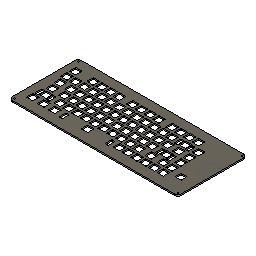
middle (Autodesk Fusion 360 design; units mm, degrees)
part number: 2026-03-14-23-22-41-149
Autodesk Fusion 360 part; units mm, degrees
(part 1 of 2)
sketch "Sketch1" plane through (0, 0, 0) normal (0, 0, 1) x (1, 0, 0)
  line L0 (-139.2143, 66.4682) -> (-126.2143, 66.4682)
  line L1 (-139.2143, 52.4682) -> (-126.2143, 52.4682)
  line L2 (-139.7143, 65.9682) -> (-139.7143, 52.9682)
  line L3 (-125.7143, 65.9682) -> (-125.7143, 52.9682)
  arc A0 (-139.2143, 66.4682) -> (-139.7143, 65.9682) centre (-139.2143, 65.9682) ccw
  arc A1 (-125.7143, 65.9682) -> (-126.2143, 66.4682) centre (-126.2143, 65.9682) ccw
  arc A2 (-139.7143, 52.9682) -> (-139.2143, 52.4682) centre (-139.2143, 52.9682) ccw
  arc A3 (-126.2143, 52.4682) -> (-125.7143, 52.9682) centre (-126.2143, 52.9682) ccw
  line L4 (-101.1143, 66.4682) -> (-88.1143, 66.4682)
  line L5 (-101.1143, 52.4682) -> (-88.1143, 52.4682)
  line L6 (-101.6143, 65.9682) -> (-101.6143, 52.9682)
  line L7 (-87.6143, 65.9682) -> (-87.6143, 52.9682)
  arc A4 (-101.1143, 66.4682) -> (-101.6143, 65.9682) centre (-101.1143, 65.9682) ccw
  arc A5 (-87.6143, 65.9682) -> (-88.1143, 66.4682) centre (-88.1143, 65.9682) ccw
  arc A6 (-101.6143, 52.9682) -> (-101.1143, 52.4682) centre (-101.1143, 52.9682) ccw
  arc A7 (-88.1143, 52.4682) -> (-87.6143, 52.9682) centre (-88.1143, 52.9682) ccw
  line L8 (-82.0643, 66.4682) -> (-69.0643, 66.4682)
  line L9 (-82.0643, 52.4682) -> (-69.0643, 52.4682)
  line L10 (-82.5643, 65.9682) -> (-82.5643, 52.9682)
  line L11 (-68.5643, 65.9682) -> (-68.5643, 52.9682)
  arc A8 (-82.0643, 66.4682) -> (-82.5643, 65.9682) centre (-82.0643, 65.9682) ccw
  arc A9 (-68.5643, 65.9682) -> (-69.0643, 66.4682) centre (-69.0643, 65.9682) ccw
  arc A10 (-82.5643, 52.9682) -> (-82.0643, 52.4682) centre (-82.0643, 52.9682) ccw
  arc A11 (-69.0643, 52.4682) -> (-68.5643, 52.9682) centre (-69.0643, 52.9682) ccw
  line L12 (-63.0143, 66.4682) -> (-50.0143, 66.4682)
  line L13 (-63.0143, 52.4682) -> (-50.0143, 52.4682)
  line L14 (-63.5143, 65.9682) -> (-63.5143, 52.9682)
  line L15 (-49.5143, 65.9682) -> (-49.5143, 52.9682)
  arc A12 (-63.0143, 66.4682) -> (-63.5143, 65.9682) centre (-63.0143, 65.9682) ccw
  arc A13 (-49.5143, 65.9682) -> (-50.0143, 66.4682) centre (-50.0143, 65.9682) ccw
  arc A14 (-63.5143, 52.9682) -> (-63.0143, 52.4682) centre (-63.0143, 52.9682) ccw
  arc A15 (-50.0143, 52.4682) -> (-49.5143, 52.9682) centre (-50.0143, 52.9682) ccw
  line L16 (-43.9643, 66.4682) -> (-30.9643, 66.4682)
  line L17 (-43.9643, 52.4682) -> (-30.9643, 52.4682)
  line L18 (-44.4643, 65.9682) -> (-44.4643, 52.9682)
  line L19 (-30.4643, 65.9682) -> (-30.4643, 52.9682)
  arc A16 (-43.9643, 66.4682) -> (-44.4643, 65.9682) centre (-43.9643, 65.9682) ccw
  arc A17 (-30.4643, 65.9682) -> (-30.9643, 66.4682) centre (-30.9643, 65.9682) ccw
  arc A18 (-44.4643, 52.9682) -> (-43.9643, 52.4682) centre (-43.9643, 52.9682) ccw
  arc A19 (-30.9643, 52.4682) -> (-30.4643, 52.9682) centre (-30.9643, 52.9682) ccw
  line L20 (-15.3893, 66.4682) -> (-2.3893, 66.4682)
  line L21 (-15.3893, 52.4682) -> (-2.3893, 52.4682)
  line L22 (-15.8893, 65.9682) -> (-15.8893, 52.9682)
  line L23 (-1.8893, 65.9682) -> (-1.8893, 52.9682)
  arc A20 (-15.3893, 66.4682) -> (-15.8893, 65.9682) centre (-15.3893, 65.9682) ccw
  arc A21 (-1.8893, 65.9682) -> (-2.3893, 66.4682) centre (-2.3893, 65.9682) ccw
  arc A22 (-15.8893, 52.9682) -> (-15.3893, 52.4682) centre (-15.3893, 52.9682) ccw
  arc A23 (-2.3893, 52.4682) -> (-1.8893, 52.9682) centre (-2.3893, 52.9682) ccw
  line L24 (3.6607, 66.4682) -> (16.6607, 66.4682)
  line L25 (3.6607, 52.4682) -> (16.6607, 52.4682)
  line L26 (3.1607, 65.9682) -> (3.1607, 52.9682)
  line L27 (17.1607, 65.9682) -> (17.1607, 52.9682)
  arc A24 (3.6607, 66.4682) -> (3.1607, 65.9682) centre (3.6607, 65.9682) ccw
  arc A25 (17.1607, 65.9682) -> (16.6607, 66.4682) centre (16.6607, 65.9682) ccw
  arc A26 (3.1607, 52.9682) -> (3.6607, 52.4682) centre (3.6607, 52.9682) ccw
  arc A27 (16.6607, 52.4682) -> (17.1607, 52.9682) centre (16.6607, 52.9682) ccw
  line L28 (22.7107, 66.4682) -> (35.7107, 66.4682)
  line L29 (22.7107, 52.4682) -> (35.7107, 52.4682)
  line L30 (22.2107, 65.9682) -> (22.2107, 52.9682)
  line L31 (36.2107, 65.9682) -> (36.2107, 52.9682)
  arc A28 (22.7107, 66.4682) -> (22.2107, 65.9682) centre (22.7107, 65.9682) ccw
  arc A29 (36.2107, 65.9682) -> (35.7107, 66.4682) centre (35.7107, 65.9682) ccw
  arc A30 (22.2107, 52.9682) -> (22.7107, 52.4682) centre (22.7107, 52.9682) ccw
  arc A31 (35.7107, 52.4682) -> (36.2107, 52.9682) centre (35.7107, 52.9682) ccw
  line L32 (41.7607, 66.4682) -> (54.7607, 66.4682)
  line L33 (41.7607, 52.4682) -> (54.7607, 52.4682)
  line L34 (41.2607, 65.9682) -> (41.2607, 52.9682)
  line L35 (55.2607, 65.9682) -> (55.2607, 52.9682)
  arc A32 (41.7607, 66.4682) -> (41.2607, 65.9682) centre (41.7607, 65.9682) ccw
  arc A33 (55.2607, 65.9682) -> (54.7607, 66.4682) centre (54.7607, 65.9682) ccw
  arc A34 (41.2607, 52.9682) -> (41.7607, 52.4682) centre (41.7607, 52.9682) ccw
  arc A35 (54.7607, 52.4682) -> (55.2607, 52.9682) centre (54.7607, 52.9682) ccw
  line L36 (70.3357, 66.4682) -> (83.3357, 66.4682)
  line L37 (70.3357, 52.4682) -> (83.3357, 52.4682)
  line L38 (69.8357, 65.9682) -> (69.8357, 52.9682)
  line L39 (83.8357, 65.9682) -> (83.8357, 52.9682)
  arc A36 (70.3357, 66.4682) -> (69.8357, 65.9682) centre (70.3357, 65.9682) ccw
  arc A37 (83.8357, 65.9682) -> (83.3357, 66.4682) centre (83.3357, 65.9682) ccw
  arc A38 (69.8357, 52.9682) -> (70.3357, 52.4682) centre (70.3357, 52.9682) ccw
  arc A39 (83.3357, 52.4682) -> (83.8357, 52.9682) centre (83.3357, 52.9682) ccw
  line L40 (89.3857, 66.4682) -> (102.3857, 66.4682)
  line L41 (89.3857, 52.4682) -> (102.3857, 52.4682)
  line L42 (88.8857, 65.9682) -> (88.8857, 52.9682)
  line L43 (102.8857, 65.9682) -> (102.8857, 52.9682)
  arc A40 (89.3857, 66.4682) -> (88.8857, 65.9682) centre (89.3857, 65.9682) ccw
  arc A41 (102.8857, 65.9682) -> (102.3857, 66.4682) centre (102.3857, 65.9682) ccw
  arc A42 (88.8857, 52.9682) -> (89.3857, 52.4682) centre (89.3857, 52.9682) ccw
  arc A43 (102.3857, 52.4682) -> (102.8857, 52.9682) centre (102.3857, 52.9682) ccw
  line L44 (108.4357, 66.4682) -> (121.4357, 66.4682)
  line L45 (108.4357, 52.4682) -> (121.4357, 52.4682)
  line L46 (107.9357, 65.9682) -> (107.9357, 52.9682)
  line L47 (121.9357, 65.9682) -> (121.9357, 52.9682)
  arc A44 (108.4357, 66.4682) -> (107.9357, 65.9682) centre (108.4357, 65.9682) ccw
  arc A45 (121.9357, 65.9682) -> (121.4357, 66.4682) centre (121.4357, 65.9682) ccw
  arc A46 (107.9357, 52.9682) -> (108.4357, 52.4682) centre (108.4357, 52.9682) ccw
  arc A47 (121.4357, 52.4682) -> (121.9357, 52.9682) centre (121.4357, 52.9682) ccw
  line L48 (127.4857, 66.4682) -> (140.4857, 66.4682)
  line L49 (127.4857, 52.4682) -> (140.4857, 52.4682)
  line L50 (126.9857, 65.9682) -> (126.9857, 52.9682)
  line L51 (140.9857, 65.9682) -> (140.9857, 52.9682)
  arc A48 (127.4857, 66.4682) -> (126.9857, 65.9682) centre (127.4857, 65.9682) ccw
  arc A49 (140.9857, 65.9682) -> (140.4857, 66.4682) centre (140.4857, 65.9682) ccw
  arc A50 (126.9857, 52.9682) -> (127.4857, 52.4682) centre (127.4857, 52.9682) ccw
  arc A51 (140.4857, 52.4682) -> (140.9857, 52.9682) centre (140.4857, 52.9682) ccw
  line L52 (-139.2143, 47.4182) -> (-126.2143, 47.4182)
  line L53 (-139.2143, 33.4182) -> (-126.2143, 33.4182)
  line L54 (-139.7143, 46.9182) -> (-139.7143, 33.9182)
  line L55 (-125.7143, 46.9182) -> (-125.7143, 33.9182)
  arc A52 (-139.2143, 47.4182) -> (-139.7143, 46.9182) centre (-139.2143, 46.9182) ccw
  arc A53 (-125.7143, 46.9182) -> (-126.2143, 47.4182) centre (-126.2143, 46.9182) ccw
  arc A54 (-139.7143, 33.9182) -> (-139.2143, 33.4182) centre (-139.2143, 33.9182) ccw
  arc A55 (-126.2143, 33.4182) -> (-125.7143, 33.9182) centre (-126.2143, 33.9182) ccw
  line L56 (-120.1643, 47.4182) -> (-107.1643, 47.4182)
  line L57 (-120.1643, 33.4182) -> (-107.1643, 33.4182)
  line L58 (-120.6643, 46.9182) -> (-120.6643, 33.9182)
  line L59 (-106.6643, 46.9182) -> (-106.6643, 33.9182)
  arc A56 (-120.1643, 47.4182) -> (-120.6643, 46.9182) centre (-120.1643, 46.9182) ccw
  arc A57 (-106.6643, 46.9182) -> (-107.1643, 47.4182) centre (-107.1643, 46.9182) ccw
  arc A58 (-120.6643, 33.9182) -> (-120.1643, 33.4182) centre (-120.1643, 33.9182) ccw
  arc A59 (-107.1643, 33.4182) -> (-106.6643, 33.9182) centre (-107.1643, 33.9182) ccw
  line L60 (-101.1143, 47.4182) -> (-88.1143, 47.4182)
  line L61 (-101.1143, 33.4182) -> (-88.1143, 33.4182)
  line L62 (-101.6143, 46.9182) -> (-101.6143, 33.9182)
  line L63 (-87.6143, 46.9182) -> (-87.6143, 33.9182)
  arc A60 (-101.1143, 47.4182) -> (-101.6143, 46.9182) centre (-101.1143, 46.9182) ccw
  arc A61 (-87.6143, 46.9182) -> (-88.1143, 47.4182) centre (-88.1143, 46.9182) ccw
  arc A62 (-101.6143, 33.9182) -> (-101.1143, 33.4182) centre (-101.1143, 33.9182) ccw
  arc A63 (-88.1143, 33.4182) -> (-87.6143, 33.9182) centre (-88.1143, 33.9182) ccw
  line L64 (-82.0643, 47.4182) -> (-69.0643, 47.4182)
  line L65 (-82.0643, 33.4182) -> (-69.0643, 33.4182)
  line L66 (-82.5643, 46.9182) -> (-82.5643, 33.9182)
  line L67 (-68.5643, 46.9182) -> (-68.5643, 33.9182)
  arc A64 (-82.0643, 47.4182) -> (-82.5643, 46.9182) centre (-82.0643, 46.9182) ccw
  arc A65 (-68.5643, 46.9182) -> (-69.0643, 47.4182) centre (-69.0643, 46.9182) ccw
  arc A66 (-82.5643, 33.9182) -> (-82.0643, 33.4182) centre (-82.0643, 33.9182) ccw
  arc A67 (-69.0643, 33.4182) -> (-68.5643, 33.9182) centre (-69.0643, 33.9182) ccw
  line L68 (-63.0143, 47.4182) -> (-50.0143, 47.4182)
  line L69 (-63.0143, 33.4182) -> (-50.0143, 33.4182)
  line L70 (-63.5143, 46.9182) -> (-63.5143, 33.9182)
  line L71 (-49.5143, 46.9182) -> (-49.5143, 33.9182)
  arc A68 (-63.0143, 47.4182) -> (-63.5143, 46.9182) centre (-63.0143, 46.9182) ccw
  arc A69 (-49.5143, 46.9182) -> (-50.0143, 47.4182) centre (-50.0143, 46.9182) ccw
  arc A70 (-63.5143, 33.9182) -> (-63.0143, 33.4182) centre (-63.0143, 33.9182) ccw
  arc A71 (-50.0143, 33.4182) -> (-49.5143, 33.9182) centre (-50.0143, 33.9182) ccw
  line L72 (-43.9643, 47.4182) -> (-30.9643, 47.4182)
  line L73 (-43.9643, 33.4182) -> (-30.9643, 33.4182)
  line L74 (-44.4643, 46.9182) -> (-44.4643, 33.9182)
  line L75 (-30.4643, 46.9182) -> (-30.4643, 33.9182)
  arc A72 (-43.9643, 47.4182) -> (-44.4643, 46.9182) centre (-43.9643, 46.9182) ccw
  arc A73 (-30.4643, 46.9182) -> (-30.9643, 47.4182) centre (-30.9643, 46.9182) ccw
  arc A74 (-44.4643, 33.9182) -> (-43.9643, 33.4182) centre (-43.9643, 33.9182) ccw
  arc A75 (-30.9643, 33.4182) -> (-30.4643, 33.9182) centre (-30.9643, 33.9182) ccw
  line L76 (-24.9143, 47.4182) -> (-11.9143, 47.4182)
  line L77 (-24.9143, 33.4182) -> (-11.9143, 33.4182)
  line L78 (-25.4143, 46.9182) -> (-25.4143, 33.9182)
  line L79 (-11.4143, 46.9182) -> (-11.4143, 33.9182)
  arc A76 (-24.9143, 47.4182) -> (-25.4143, 46.9182) centre (-24.9143, 46.9182) ccw
  arc A77 (-11.4143, 46.9182) -> (-11.9143, 47.4182) centre (-11.9143, 46.9182) ccw
  arc A78 (-25.4143, 33.9182) -> (-24.9143, 33.4182) centre (-24.9143, 33.9182) ccw
  arc A79 (-11.9143, 33.4182) -> (-11.4143, 33.9182) centre (-11.9143, 33.9182) ccw
  line L80 (-5.8643, 47.4182) -> (7.1357, 47.4182)
  line L81 (-5.8643, 33.4182) -> (7.1357, 33.4182)
  line L82 (-6.3643, 46.9182) -> (-6.3643, 33.9182)
  line L83 (7.6357, 46.9182) -> (7.6357, 33.9182)
  arc A80 (-5.8643, 47.4182) -> (-6.3643, 46.9182) centre (-5.8643, 46.9182) ccw
  arc A81 (7.6357, 46.9182) -> (7.1357, 47.4182) centre (7.1357, 46.9182) ccw
  arc A82 (-6.3643, 33.9182) -> (-5.8643, 33.4182) centre (-5.8643, 33.9182) ccw
  arc A83 (7.1357, 33.4182) -> (7.6357, 33.9182) centre (7.1357, 33.9182) ccw
  line L84 (13.1857, 47.4182) -> (26.1857, 47.4182)
  line L85 (13.1857, 33.4182) -> (26.1857, 33.4182)
  line L86 (12.6857, 46.9182) -> (12.6857, 33.9182)
  line L87 (26.6857, 46.9182) -> (26.6857, 33.9182)
  arc A84 (13.1857, 47.4182) -> (12.6857, 46.9182) centre (13.1857, 46.9182) ccw
  arc A85 (26.6857, 46.9182) -> (26.1857, 47.4182) centre (26.1857, 46.9182) ccw
  arc A86 (12.6857, 33.9182) -> (13.1857, 33.4182) centre (13.1857, 33.9182) ccw
  arc A87 (26.1857, 33.4182) -> (26.6857, 33.9182) centre (26.1857, 33.9182) ccw
  line L88 (32.2357, 47.4182) -> (45.2357, 47.4182)
  line L89 (32.2357, 33.4182) -> (45.2357, 33.4182)
  line L90 (31.7357, 46.9182) -> (31.7357, 33.9182)
  line L91 (45.7357, 46.9182) -> (45.7357, 33.9182)
  arc A88 (32.2357, 47.4182) -> (31.7357, 46.9182) centre (32.2357, 46.9182) ccw
  arc A89 (45.7357, 46.9182) -> (45.2357, 47.4182) centre (45.2357, 46.9182) ccw
  arc A90 (31.7357, 33.9182) -> (32.2357, 33.4182) centre (32.2357, 33.9182) ccw
  arc A91 (45.2357, 33.4182) -> (45.7357, 33.9182) centre (45.2357, 33.9182) ccw
  line L92 (51.2857, 47.4182) -> (64.2857, 47.4182)
  line L93 (51.2857, 33.4182) -> (64.2857, 33.4182)
  line L94 (50.7857, 46.9182) -> (50.7857, 33.9182)
  line L95 (64.7857, 46.9182) -> (64.7857, 33.9182)
  arc A92 (51.2857, 47.4182) -> (50.7857, 46.9182) centre (51.2857, 46.9182) ccw
  arc A93 (64.7857, 46.9182) -> (64.2857, 47.4182) centre (64.2857, 46.9182) ccw
  arc A94 (50.7857, 33.9182) -> (51.2857, 33.4182) centre (51.2857, 33.9182) ccw
  arc A95 (64.2857, 33.4182) -> (64.7857, 33.9182) centre (64.2857, 33.9182) ccw
  line L96 (70.3357, 47.4182) -> (83.3357, 47.4182)
  line L97 (70.3357, 33.4182) -> (83.3357, 33.4182)
  line L98 (69.8357, 46.9182) -> (69.8357, 33.9182)
  line L99 (83.8357, 46.9182) -> (83.8357, 33.9182)
  arc A96 (70.3357, 47.4182) -> (69.8357, 46.9182) centre (70.3357, 46.9182) ccw
  arc A97 (83.8357, 46.9182) -> (83.3357, 47.4182) centre (83.3357, 46.9182) ccw
  arc A98 (69.8357, 33.9182) -> (70.3357, 33.4182) centre (70.3357, 33.9182) ccw
  arc A99 (83.3357, 33.4182) -> (83.8357, 33.9182) centre (83.3357, 33.9182) ccw
  line L100 (89.3857, 47.4182) -> (102.3857, 47.4182)
  line L101 (89.3857, 33.4182) -> (102.3857, 33.4182)
  line L102 (88.8857, 46.9182) -> (88.8857, 33.9182)
  line L103 (102.8857, 46.9182) -> (102.8857, 33.9182)
  arc A100 (89.3857, 47.4182) -> (88.8857, 46.9182) centre (89.3857, 46.9182) ccw
  arc A101 (102.8857, 46.9182) -> (102.3857, 47.4182) centre (102.3857, 46.9182) ccw
  arc A102 (88.8857, 33.9182) -> (89.3857, 33.4182) centre (89.3857, 33.9182) ccw
  arc A103 (102.3857, 33.4182) -> (102.8857, 33.9182) centre (102.3857, 33.9182) ccw
  line L104 (117.9607, 47.4182) -> (130.9607, 47.4182)
  line L105 (117.9607, 33.4182) -> (130.9607, 33.4182)
  line L106 (117.4607, 46.9182) -> (117.4607, 33.9182)
  line L107 (131.4607, 46.9182) -> (131.4607, 33.9182)
  arc A104 (117.9607, 47.4182) -> (117.4607, 46.9182) centre (117.9607, 46.9182) ccw
  arc A105 (131.4607, 46.9182) -> (130.9607, 47.4182) centre (130.9607, 46.9182) ccw
  arc A106 (117.4607, 33.9182) -> (117.9607, 33.4182) centre (117.9607, 33.9182) ccw
  arc A107 (130.9607, 33.4182) -> (131.4607, 33.9182) centre (130.9607, 33.9182) ccw
  line L108 (109.5227, 46.4182) -> (115.5227, 46.4182)
  line L109 (109.5227, 31.4182) -> (115.5227, 31.4182)
  line L110 (109.0227, 45.9182) -> (109.0227, 31.9182)
  line L111 (116.0227, 45.9182) -> (116.0227, 31.9182)
  arc A108 (109.5227, 46.4182) -> (109.0227, 45.9182) centre (109.5227, 45.9182) ccw
  arc A109 (116.0227, 45.9182) -> (115.5227, 46.4182) centre (115.5227, 45.9182) ccw
  arc A110 (109.0227, 31.9182) -> (109.5227, 31.4182) centre (109.5227, 31.9182) ccw
  arc A111 (115.5227, 31.4182) -> (116.0227, 31.9182) centre (115.5227, 31.9182) ccw
  line L112 (133.3987, 46.4182) -> (139.3987, 46.4182)
  line L113 (133.3987, 31.4182) -> (139.3987, 31.4182)
  line L114 (132.8987, 45.9182) -> (132.8987, 31.9182)
  line L115 (139.8987, 45.9182) -> (139.8987, 31.9182)
  arc A112 (133.3987, 46.4182) -> (132.8987, 45.9182) centre (133.3987, 45.9182) ccw
  arc A113 (139.8987, 45.9182) -> (139.3987, 46.4182) centre (139.3987, 45.9182) ccw
  arc A114 (132.8987, 31.9182) -> (133.3987, 31.4182) centre (133.3987, 31.9182) ccw
  arc A115 (139.3987, 31.4182) -> (139.8987, 31.9182) centre (139.3987, 31.9182) ccw
  line L116 (146.5357, 47.4182) -> (159.5357, 47.4182)
  line L117 (146.5357, 33.4182) -> (159.5357, 33.4182)
  line L118 (146.0357, 46.9182) -> (146.0357, 33.9182)
  line L119 (160.0357, 46.9182) -> (160.0357, 33.9182)
  arc A116 (146.5357, 47.4182) -> (146.0357, 46.9182) centre (146.5357, 46.9182) ccw
  arc A117 (160.0357, 46.9182) -> (159.5357, 47.4182) centre (159.5357, 46.9182) ccw
  arc A118 (146.0357, 33.9182) -> (146.5357, 33.4182) centre (146.5357, 33.9182) ccw
  arc A119 (159.5357, 33.4182) -> (160.0357, 33.9182) centre (159.5357, 33.9182) ccw
  line L120 (-134.4518, 28.3682) -> (-121.4518, 28.3682)
  line L121 (-134.4518, 14.3682) -> (-121.4518, 14.3682)
  line L122 (-134.9518, 27.8682) -> (-134.9518, 14.8682)
  line L123 (-120.9518, 27.8682) -> (-120.9518, 14.8682)
  arc A120 (-134.4518, 28.3682) -> (-134.9518, 27.8682) centre (-134.4518, 27.8682) ccw
  arc A121 (-120.9518, 27.8682) -> (-121.4518, 28.3682) centre (-121.4518, 27.8682) ccw
  arc A122 (-134.9518, 14.8682) -> (-134.4518, 14.3682) centre (-134.4518, 14.8682) ccw
  arc A123 (-121.4518, 14.3682) -> (-120.9518, 14.8682) centre (-121.4518, 14.8682) ccw
  line L124 (-110.6393, 28.3682) -> (-97.6393, 28.3682)
  line L125 (-110.6393, 14.3682) -> (-97.6393, 14.3682)
  line L126 (-111.1393, 27.8682) -> (-111.1393, 14.8682)
  line L127 (-97.1393, 27.8682) -> (-97.1393, 14.8682)
  arc A124 (-110.6393, 28.3682) -> (-111.1393, 27.8682) centre (-110.6393, 27.8682) ccw
  arc A125 (-97.1393, 27.8682) -> (-97.6393, 28.3682) centre (-97.6393, 27.8682) ccw
  arc A126 (-111.1393, 14.8682) -> (-110.6393, 14.3682) centre (-110.6393, 14.8682) ccw
  arc A127 (-97.6393, 14.3682) -> (-97.1393, 14.8682) centre (-97.6393, 14.8682) ccw
  line L128 (-91.5893, 28.3682) -> (-78.5893, 28.3682)
  line L129 (-91.5893, 14.3682) -> (-78.5893, 14.3682)
  line L130 (-92.0893, 27.8682) -> (-92.0893, 14.8682)
  line L131 (-78.0893, 27.8682) -> (-78.0893, 14.8682)
  arc A128 (-91.5893, 28.3682) -> (-92.0893, 27.8682) centre (-91.5893, 27.8682) ccw
  arc A129 (-78.0893, 27.8682) -> (-78.5893, 28.3682) centre (-78.5893, 27.8682) ccw
  arc A130 (-92.0893, 14.8682) -> (-91.5893, 14.3682) centre (-91.5893, 14.8682) ccw
  arc A131 (-78.5893, 14.3682) -> (-78.0893, 14.8682) centre (-78.5893, 14.8682) ccw
  line L132 (-72.5393, 28.3682) -> (-59.5393, 28.3682)
  line L133 (-72.5393, 14.3682) -> (-59.5393, 14.3682)
  line L134 (-73.0393, 27.8682) -> (-73.0393, 14.8682)
  line L135 (-59.0393, 27.8682) -> (-59.0393, 14.8682)
  arc A132 (-72.5393, 28.3682) -> (-73.0393, 27.8682) centre (-72.5393, 27.8682) ccw
  arc A133 (-59.0393, 27.8682) -> (-59.5393, 28.3682) centre (-59.5393, 27.8682) ccw
  arc A134 (-73.0393, 14.8682) -> (-72.5393, 14.3682) centre (-72.5393, 14.8682) ccw
  arc A135 (-59.5393, 14.3682) -> (-59.0393, 14.8682) centre (-59.5393, 14.8682) ccw
  line L136 (-53.4893, 28.3682) -> (-40.4893, 28.3682)
  line L137 (-53.4893, 14.3682) -> (-40.4893, 14.3682)
  line L138 (-53.9893, 27.8682) -> (-53.9893, 14.8682)
  line L139 (-39.9893, 27.8682) -> (-39.9893, 14.8682)
  arc A136 (-53.4893, 28.3682) -> (-53.9893, 27.8682) centre (-53.4893, 27.8682) ccw
  arc A137 (-39.9893, 27.8682) -> (-40.4893, 28.3682) centre (-40.4893, 27.8682) ccw
  arc A138 (-53.9893, 14.8682) -> (-53.4893, 14.3682) centre (-53.4893, 14.8682) ccw
  arc A139 (-40.4893, 14.3682) -> (-39.9893, 14.8682) centre (-40.4893, 14.8682) ccw
  line L140 (-34.4393, 28.3682) -> (-21.4393, 28.3682)
  line L141 (-34.4393, 14.3682) -> (-21.4393, 14.3682)
  line L142 (-34.9393, 27.8682) -> (-34.9393, 14.8682)
  line L143 (-20.9393, 27.8682) -> (-20.9393, 14.8682)
  arc A140 (-34.4393, 28.3682) -> (-34.9393, 27.8682) centre (-34.4393, 27.8682) ccw
  arc A141 (-20.9393, 27.8682) -> (-21.4393, 28.3682) centre (-21.4393, 27.8682) ccw
  arc A142 (-34.9393, 14.8682) -> (-34.4393, 14.3682) centre (-34.4393, 14.8682) ccw
  arc A143 (-21.4393, 14.3682) -> (-20.9393, 14.8682) centre (-21.4393, 14.8682) ccw
  line L144 (-15.3893, 28.3682) -> (-2.3893, 28.3682)
  line L145 (-15.3893, 14.3682) -> (-2.3893, 14.3682)
  line L146 (-15.8893, 27.8682) -> (-15.8893, 14.8682)
  line L147 (-1.8893, 27.8682) -> (-1.8893, 14.8682)
  arc A144 (-15.3893, 28.3682) -> (-15.8893, 27.8682) centre (-15.3893, 27.8682) ccw
  arc A145 (-1.8893, 27.8682) -> (-2.3893, 28.3682) centre (-2.3893, 27.8682) ccw
  arc A146 (-15.8893, 14.8682) -> (-15.3893, 14.3682) centre (-15.3893, 14.8682) ccw
  arc A147 (-2.3893, 14.3682) -> (-1.8893, 14.8682) centre (-2.3893, 14.8682) ccw
  line L148 (3.6607, 28.3682) -> (16.6607, 28.3682)
  line L149 (3.6607, 14.3682) -> (16.6607, 14.3682)
  line L150 (3.1607, 27.8682) -> (3.1607, 14.8682)
  line L151 (17.1607, 27.8682) -> (17.1607, 14.8682)
  arc A148 (3.6607, 28.3682) -> (3.1607, 27.8682) centre (3.6607, 27.8682) ccw
  arc A149 (17.1607, 27.8682) -> (16.6607, 28.3682) centre (16.6607, 27.8682) ccw
  arc A150 (3.1607, 14.8682) -> (3.6607, 14.3682) centre (3.6607, 14.8682) ccw
  arc A151 (16.6607, 14.3682) -> (17.1607, 14.8682) centre (16.6607, 14.8682) ccw
  line L152 (22.7107, 28.3682) -> (35.7107, 28.3682)
  line L153 (22.7107, 14.3682) -> (35.7107, 14.3682)
  line L154 (22.2107, 27.8682) -> (22.2107, 14.8682)
  line L155 (36.2107, 27.8682) -> (36.2107, 14.8682)
  arc A152 (22.7107, 28.3682) -> (22.2107, 27.8682) centre (22.7107, 27.8682) ccw
  arc A153 (36.2107, 27.8682) -> (35.7107, 28.3682) centre (35.7107, 27.8682) ccw
  arc A154 (22.2107, 14.8682) -> (22.7107, 14.3682) centre (22.7107, 14.8682) ccw
  arc A155 (35.7107, 14.3682) -> (36.2107, 14.8682) centre (35.7107, 14.8682) ccw
  line L156 (41.7607, 28.3682) -> (54.7607, 28.3682)
  line L157 (41.7607, 14.3682) -> (54.7607, 14.3682)
  line L158 (41.2607, 27.8682) -> (41.2607, 14.8682)
  line L159 (55.2607, 27.8682) -> (55.2607, 14.8682)
  arc A156 (41.7607, 28.3682) -> (41.2607, 27.8682) centre (41.7607, 27.8682) ccw
  arc A157 (55.2607, 27.8682) -> (54.7607, 28.3682) centre (54.7607, 27.8682) ccw
  arc A158 (41.2607, 14.8682) -> (41.7607, 14.3682) centre (41.7607, 14.8682) ccw
  arc A159 (54.7607, 14.3682) -> (55.2607, 14.8682) centre (54.7607, 14.8682) ccw
  line L160 (60.8107, 28.3682) -> (73.8107, 28.3682)
  line L161 (60.8107, 14.3682) -> (73.8107, 14.3682)
  line L162 (60.3107, 27.8682) -> (60.3107, 14.8682)
  line L163 (74.3107, 27.8682) -> (74.3107, 14.8682)
  arc A160 (60.8107, 28.3682) -> (60.3107, 27.8682) centre (60.8107, 27.8682) ccw
  arc A161 (74.3107, 27.8682) -> (73.8107, 28.3682) centre (73.8107, 27.8682) ccw
  arc A162 (60.3107, 14.8682) -> (60.8107, 14.3682) centre (60.8107, 14.8682) ccw
  arc A163 (73.8107, 14.3682) -> (74.3107, 14.8682) centre (73.8107, 14.8682) ccw
  line L164 (79.8607, 28.3682) -> (92.8607, 28.3682)
  line L165 (79.8607, 14.3682) -> (92.8607, 14.3682)
  line L166 (79.3607, 27.8682) -> (79.3607, 14.8682)
  line L167 (93.3607, 27.8682) -> (93.3607, 14.8682)
  arc A164 (79.8607, 28.3682) -> (79.3607, 27.8682) centre (79.8607, 27.8682) ccw
  arc A165 (93.3607, 27.8682) -> (92.8607, 28.3682) centre (92.8607, 27.8682) ccw
  arc A166 (79.3607, 14.8682) -> (79.8607, 14.3682) centre (79.8607, 14.8682) ccw
  arc A167 (92.8607, 14.3682) -> (93.3607, 14.8682) centre (92.8607, 14.8682) ccw
  line L168 (98.9107, 28.3682) -> (111.9107, 28.3682)
  line L169 (98.9107, 14.3682) -> (111.9107, 14.3682)
  line L170 (98.4107, 27.8682) -> (98.4107, 14.8682)
  line L171 (112.4107, 27.8682) -> (112.4107, 14.8682)
  arc A168 (98.9107, 28.3682) -> (98.4107, 27.8682) centre (98.9107, 27.8682) ccw
  arc A169 (112.4107, 27.8682) -> (111.9107, 28.3682) centre (111.9107, 27.8682) ccw
  arc A170 (98.4107, 14.8682) -> (98.9107, 14.3682) centre (98.9107, 14.8682) ccw
  arc A171 (111.9107, 14.3682) -> (112.4107, 14.8682) centre (111.9107, 14.8682) ccw
  line L172 (122.7232, 28.3682) -> (135.7232, 28.3682)
  line L173 (122.7232, 14.3682) -> (135.7232, 14.3682)
  line L174 (122.2232, 27.8682) -> (122.2232, 14.8682)
  line L175 (136.2232, 27.8682) -> (136.2232, 14.8682)
  arc A172 (122.7232, 28.3682) -> (122.2232, 27.8682) centre (122.7232, 27.8682) ccw
  arc A173 (136.2232, 27.8682) -> (135.7232, 28.3682) centre (135.7232, 27.8682) ccw
  arc A174 (122.2232, 14.8682) -> (122.7232, 14.3682) centre (122.7232, 14.8682) ccw
  arc A175 (135.7232, 14.3682) -> (136.2232, 14.8682) centre (135.7232, 14.8682) ccw
  line L176 (146.5357, 28.3682) -> (159.5357, 28.3682)
  line L177 (146.5357, 14.3682) -> (159.5357, 14.3682)
  line L178 (146.0357, 27.8682) -> (146.0357, 14.8682)
  line L179 (160.0357, 27.8682) -> (160.0357, 14.8682)
  arc A176 (146.5357, 28.3682) -> (146.0357, 27.8682) centre (146.5357, 27.8682) ccw
  arc A177 (160.0357, 27.8682) -> (159.5357, 28.3682) centre (159.5357, 27.8682) ccw
  arc A178 (146.0357, 14.8682) -> (146.5357, 14.3682) centre (146.5357, 14.8682) ccw
  arc A179 (159.5357, 14.3682) -> (160.0357, 14.8682) centre (159.5357, 14.8682) ccw
  line L180 (-132.0706, 9.3182) -> (-119.0706, 9.3182)
  line L181 (-132.0706, -4.6818) -> (-119.0706, -4.6818)
  line L182 (-132.5706, 8.8182) -> (-132.5706, -4.1818)
  line L183 (-118.5706, 8.8182) -> (-118.5706, -4.1818)
  arc A180 (-132.0706, 9.3182) -> (-132.5706, 8.8182) centre (-132.0706, 8.8182) ccw
  arc A181 (-118.5706, 8.8182) -> (-119.0706, 9.3182) centre (-119.0706, 8.8182) ccw
  arc A182 (-132.5706, -4.1818) -> (-132.0706, -4.6818) centre (-132.0706, -4.1818) ccw
  arc A183 (-119.0706, -4.6818) -> (-118.5706, -4.1818) centre (-119.0706, -4.1818) ccw
  line L184 (-105.8768, 9.3182) -> (-92.8768, 9.3182)
  line L185 (-105.8768, -4.6818) -> (-92.8768, -4.6818)
  line L186 (-106.3768, 8.8182) -> (-106.3768, -4.1818)
  line L187 (-92.3768, 8.8182) -> (-92.3768, -4.1818)
  arc A184 (-105.8768, 9.3182) -> (-106.3768, 8.8182) centre (-105.8768, 8.8182) ccw
  arc A185 (-92.3768, 8.8182) -> (-92.8768, 9.3182) centre (-92.8768, 8.8182) ccw
  arc A186 (-106.3768, -4.1818) -> (-105.8768, -4.6818) centre (-105.8768, -4.1818) ccw
  arc A187 (-92.8768, -4.6818) -> (-92.3768, -4.1818) centre (-92.8768, -4.1818) ccw
  line L188 (-86.8268, 9.3182) -> (-73.8268, 9.3182)
  line L189 (-86.8268, -4.6818) -> (-73.8268, -4.6818)
  line L190 (-87.3268, 8.8182) -> (-87.3268, -4.1818)
  line L191 (-73.3268, 8.8182) -> (-73.3268, -4.1818)
  arc A188 (-86.8268, 9.3182) -> (-87.3268, 8.8182) centre (-86.8268, 8.8182) ccw
  arc A189 (-73.3268, 8.8182) -> (-73.8268, 9.3182) centre (-73.8268, 8.8182) ccw
  arc A190 (-87.3268, -4.1818) -> (-86.8268, -4.6818) centre (-86.8268, -4.1818) ccw
  arc A191 (-73.8268, -4.6818) -> (-73.3268, -4.1818) centre (-73.8268, -4.1818) ccw
  line L192 (-67.7768, 9.3182) -> (-54.7768, 9.3182)
  line L193 (-67.7768, -4.6818) -> (-54.7768, -4.6818)
  line L194 (-68.2768, 8.8182) -> (-68.2768, -4.1818)
  line L195 (-54.2768, 8.8182) -> (-54.2768, -4.1818)
  arc A192 (-67.7768, 9.3182) -> (-68.2768, 8.8182) centre (-67.7768, 8.8182) ccw
  arc A193 (-54.2768, 8.8182) -> (-54.7768, 9.3182) centre (-54.7768, 8.8182) ccw
  arc A194 (-68.2768, -4.1818) -> (-67.7768, -4.6818) centre (-67.7768, -4.1818) ccw
  arc A195 (-54.7768, -4.6818) -> (-54.2768, -4.1818) centre (-54.7768, -4.1818) ccw
  line L196 (-48.7268, 9.3182) -> (-35.7268, 9.3182)
  line L197 (-48.7268, -4.6818) -> (-35.7268, -4.6818)
  line L198 (-49.2268, 8.8182) -> (-49.2268, -4.1818)
  line L199 (-35.2268, 8.8182) -> (-35.2268, -4.1818)
  arc A196 (-48.7268, 9.3182) -> (-49.2268, 8.8182) centre (-48.7268, 8.8182) ccw
  arc A197 (-35.2268, 8.8182) -> (-35.7268, 9.3182) centre (-35.7268, 8.8182) ccw
  arc A198 (-49.2268, -4.1818) -> (-48.7268, -4.6818) centre (-48.7268, -4.1818) ccw
  arc A199 (-35.7268, -4.6818) -> (-35.2268, -4.1818) centre (-35.7268, -4.1818) ccw
  line L200 (-29.6768, 9.3182) -> (-16.6768, 9.3182)
  line L201 (-29.6768, -4.6818) -> (-16.6768, -4.6818)
  line L202 (-30.1768, 8.8182) -> (-30.1768, -4.1818)
  line L203 (-16.1768, 8.8182) -> (-16.1768, -4.1818)
  arc A200 (-29.6768, 9.3182) -> (-30.1768, 8.8182) centre (-29.6768, 8.8182) ccw
  arc A201 (-16.1768, 8.8182) -> (-16.6768, 9.3182) centre (-16.6768, 8.8182) ccw
  arc A202 (-30.1768, -4.1818) -> (-29.6768, -4.6818) centre (-29.6768, -4.1818) ccw
  arc A203 (-16.6768, -4.6818) -> (-16.1768, -4.1818) centre (-16.6768, -4.1818) ccw
  line L204 (-10.6268, 9.3182) -> (2.3732, 9.3182)
  line L205 (-10.6268, -4.6818) -> (2.3732, -4.6818)
  line L206 (-11.1268, 8.8182) -> (-11.1268, -4.1818)
  line L207 (2.8732, 8.8182) -> (2.8732, -4.1818)
  arc A204 (-10.6268, 9.3182) -> (-11.1268, 8.8182) centre (-10.6268, 8.8182) ccw
  arc A205 (2.8732, 8.8182) -> (2.3732, 9.3182) centre (2.3732, 8.8182) ccw
  arc A206 (-11.1268, -4.1818) -> (-10.6268, -4.6818) centre (-10.6268, -4.1818) ccw
  arc A207 (2.3732, -4.6818) -> (2.8732, -4.1818) centre (2.3732, -4.1818) ccw
  line L208 (8.4232, 9.3182) -> (21.4232, 9.3182)
  line L209 (8.4232, -4.6818) -> (21.4232, -4.6818)
  line L210 (7.9232, 8.8182) -> (7.9232, -4.1818)
  line L211 (21.9232, 8.8182) -> (21.9232, -4.1818)
  arc A208 (8.4232, 9.3182) -> (7.9232, 8.8182) centre (8.4232, 8.8182) ccw
  arc A209 (21.9232, 8.8182) -> (21.4232, 9.3182) centre (21.4232, 8.8182) ccw
  arc A210 (7.9232, -4.1818) -> (8.4232, -4.6818) centre (8.4232, -4.1818) ccw
  arc A211 (21.4232, -4.6818) -> (21.9232, -4.1818) centre (21.4232, -4.1818) ccw
  line L212 (27.4732, 9.3182) -> (40.4732, 9.3182)
  line L213 (27.4732, -4.6818) -> (40.4732, -4.6818)
  line L214 (26.9732, 8.8182) -> (26.9732, -4.1818)
  line L215 (40.9732, 8.8182) -> (40.9732, -4.1818)
  arc A212 (27.4732, 9.3182) -> (26.9732, 8.8182) centre (27.4732, 8.8182) ccw
  arc A213 (40.9732, 8.8182) -> (40.4732, 9.3182) centre (40.4732, 8.8182) ccw
  arc A214 (26.9732, -4.1818) -> (27.4732, -4.6818) centre (27.4732, -4.1818) ccw
  arc A215 (40.4732, -4.6818) -> (40.9732, -4.1818) centre (40.4732, -4.1818) ccw
  line L216 (46.5232, 9.3182) -> (59.5232, 9.3182)
  line L217 (46.5232, -4.6818) -> (59.5232, -4.6818)
  line L218 (46.0232, 8.8182) -> (46.0232, -4.1818)
  line L219 (60.0232, 8.8182) -> (60.0232, -4.1818)
  arc A216 (46.5232, 9.3182) -> (46.0232, 8.8182) centre (46.5232, 8.8182) ccw
  arc A217 (60.0232, 8.8182) -> (59.5232, 9.3182) centre (59.5232, 8.8182) ccw
  arc A218 (46.0232, -4.1818) -> (46.5232, -4.6818) centre (46.5232, -4.1818) ccw
  arc A219 (59.5232, -4.6818) -> (60.0232, -4.1818) centre (59.5232, -4.1818) ccw
  line L220 (65.5732, 9.3182) -> (78.5732, 9.3182)
  line L221 (65.5732, -4.6818) -> (78.5732, -4.6818)
  line L222 (65.0732, 8.8182) -> (65.0732, -4.1818)
  line L223 (79.0732, 8.8182) -> (79.0732, -4.1818)
  arc A220 (65.5732, 9.3182) -> (65.0732, 8.8182) centre (65.5732, 8.8182) ccw
  arc A221 (79.0732, 8.8182) -> (78.5732, 9.3182) centre (78.5732, 8.8182) ccw
  arc A222 (65.0732, -4.1818) -> (65.5732, -4.6818) centre (65.5732, -4.1818) ccw
  arc A223 (78.5732, -4.6818) -> (79.0732, -4.1818) centre (78.5732, -4.1818) ccw
  line L224 (84.6232, 9.3182) -> (97.6232, 9.3182)
  line L225 (84.6232, -4.6818) -> (97.6232, -4.6818)
  line L226 (84.1232, 8.8182) -> (84.1232, -4.1818)
  line L227 (98.1232, 8.8182) -> (98.1232, -4.1818)
  arc A224 (84.6232, 9.3182) -> (84.1232, 8.8182) centre (84.6232, 8.8182) ccw
  arc A225 (98.1232, 8.8182) -> (97.6232, 9.3182) centre (97.6232, 8.8182) ccw
  arc A226 (84.1232, -4.1818) -> (84.6232, -4.6818) centre (84.6232, -4.1818) ccw
  arc A227 (97.6232, -4.6818) -> (98.1232, -4.1818) centre (97.6232, -4.1818) ccw
  line L228 (115.5794, 9.3182) -> (128.5794, 9.3182)
  line L229 (115.5794, -4.6818) -> (128.5794, -4.6818)
  line L230 (115.0794, 8.8182) -> (115.0794, -4.1818)
  line L231 (129.0794, 8.8182) -> (129.0794, -4.1818)
  arc A228 (115.5794, 9.3182) -> (115.0794, 8.8182) centre (115.5794, 8.8182) ccw
  arc A229 (129.0794, 8.8182) -> (128.5794, 9.3182) centre (128.5794, 8.8182) ccw
  arc A230 (115.0794, -4.1818) -> (115.5794, -4.6818) centre (115.5794, -4.1818) ccw
  arc A231 (128.5794, -4.6818) -> (129.0794, -4.1818) centre (128.5794, -4.1818) ccw
  line L232 (107.1414, 8.3182) -> (113.1414, 8.3182)
  line L233 (107.1414, -6.6818) -> (113.1414, -6.6818)
  line L234 (106.6414, 7.8182) -> (106.6414, -6.1818)
  line L235 (113.6414, 7.8182) -> (113.6414, -6.1818)
  arc A232 (107.1414, 8.3182) -> (106.6414, 7.8182) centre (107.1414, 7.8182) ccw
  arc A233 (113.6414, 7.8182) -> (113.1414, 8.3182) centre (113.1414, 7.8182) ccw
  arc A234 (106.6414, -6.1818) -> (107.1414, -6.6818) centre (107.1414, -6.1818) ccw
  arc A235 (113.1414, -6.6818) -> (113.6414, -6.1818) centre (113.1414, -6.1818) ccw
  line L236 (131.0174, 8.3182) -> (137.0174, 8.3182)
  line L237 (131.0174, -6.6818) -> (137.0174, -6.6818)
  line L238 (130.5174, 7.8182) -> (130.5174, -6.1818)
  line L239 (137.5174, 7.8182) -> (137.5174, -6.1818)
  arc A236 (131.0174, 8.3182) -> (130.5174, 7.8182) centre (131.0174, 7.8182) ccw
  arc A237 (137.5174, 7.8182) -> (137.0174, 8.3182) centre (137.0174, 7.8182) ccw
  arc A238 (130.5174, -6.1818) -> (131.0174, -6.6818) centre (131.0174, -6.1818) ccw
  arc A239 (137.0174, -6.6818) -> (137.5174, -6.1818) centre (137.0174, -6.1818) ccw
  line L240 (146.5357, 9.3182) -> (159.5357, 9.3182)
  line L241 (146.5357, -4.6818) -> (159.5357, -4.6818)
  line L242 (146.0357, 8.8182) -> (146.0357, -4.1818)
  line L243 (160.0357, 8.8182) -> (160.0357, -4.1818)
  arc A240 (146.5357, 9.3182) -> (146.0357, 8.8182) centre (146.5357, 8.8182) ccw
  arc A241 (160.0357, 8.8182) -> (159.5357, 9.3182) centre (159.5357, 8.8182) ccw
  arc A242 (146.0357, -4.1818) -> (146.5357, -4.6818) centre (146.5357, -4.1818) ccw
  arc A243 (159.5357, -4.6818) -> (160.0357, -4.1818) centre (159.5357, -4.1818) ccw
  line L244 (-127.3081, -9.7318) -> (-114.3081, -9.7318)
  line L245 (-127.3081, -23.7318) -> (-114.3081, -23.7318)
  line L246 (-127.8081, -10.2318) -> (-127.8081, -23.2318)
  line L247 (-113.8081, -10.2318) -> (-113.8081, -23.2318)
  arc A244 (-127.3081, -9.7318) -> (-127.8081, -10.2318) centre (-127.3081, -10.2318) ccw
  arc A245 (-113.8081, -10.2318) -> (-114.3081, -9.7318) centre (-114.3081, -10.2318) ccw
  arc A246 (-127.8081, -23.2318) -> (-127.3081, -23.7318) centre (-127.3081, -23.2318) ccw
  arc A247 (-114.3081, -23.7318) -> (-113.8081, -23.2318) centre (-114.3081, -23.2318) ccw
  line L248 (-135.7461, -10.7318) -> (-129.7461, -10.7318)
  line L249 (-135.7461, -25.7318) -> (-129.7461, -25.7318)
  line L250 (-136.2461, -11.2318) -> (-136.2461, -25.2318)
  line L251 (-129.2461, -11.2318) -> (-129.2461, -25.2318)
  arc A248 (-135.7461, -10.7318) -> (-136.2461, -11.2318) centre (-135.7461, -11.2318) ccw
  arc A249 (-129.2461, -11.2318) -> (-129.7461, -10.7318) centre (-129.7461, -11.2318) ccw
  arc A250 (-136.2461, -25.2318) -> (-135.7461, -25.7318) centre (-135.7461, -25.2318) ccw
  arc A251 (-129.7461, -25.7318) -> (-129.2461, -25.2318) centre (-129.7461, -25.2318) ccw
  line L252 (-111.8701, -10.7318) -> (-105.8701, -10.7318)
  line L253 (-111.8701, -25.7318) -> (-105.8701, -25.7318)
  line L254 (-112.3701, -11.2318) -> (-112.3701, -25.2318)
  line L255 (-105.3701, -11.2318) -> (-105.3701, -25.2318)
  arc A252 (-111.8701, -10.7318) -> (-112.3701, -11.2318) centre (-111.8701, -11.2318) ccw
  arc A253 (-105.3701, -11.2318) -> (-105.8701, -10.7318) centre (-105.8701, -11.2318) ccw
  arc A254 (-112.3701, -25.2318) -> (-111.8701, -25.7318) centre (-111.8701, -25.2318) ccw
  arc A255 (-105.8701, -25.7318) -> (-105.3701, -25.2318) centre (-105.8701, -25.2318) ccw
  line L256 (-96.3518, -9.7318) -> (-83.3518, -9.7318)
  line L257 (-96.3518, -23.7318) -> (-83.3518, -23.7318)
  line L258 (-96.8518, -10.2318) -> (-96.8518, -23.2318)
  line L259 (-82.8518, -10.2318) -> (-82.8518, -23.2318)
  arc A256 (-96.3518, -9.7318) -> (-96.8518, -10.2318) centre (-96.3518, -10.2318) ccw
  arc A257 (-82.8518, -10.2318) -> (-83.3518, -9.7318) centre (-83.3518, -10.2318) ccw
  arc A258 (-96.8518, -23.2318) -> (-96.3518, -23.7318) centre (-96.3518, -23.2318) ccw
  arc A259 (-83.3518, -23.7318) -> (-82.8518, -23.2318) centre (-83.3518, -23.2318) ccw
  line L260 (-77.3018, -9.7318) -> (-64.3018, -9.7318)
  line L261 (-77.3018, -23.7318) -> (-64.3018, -23.7318)
  line L262 (-77.8018, -10.2318) -> (-77.8018, -23.2318)
  line L263 (-63.8018, -10.2318) -> (-63.8018, -23.2318)
  arc A260 (-77.3018, -9.7318) -> (-77.8018, -10.2318) centre (-77.3018, -10.2318) ccw
  arc A261 (-63.8018, -10.2318) -> (-64.3018, -9.7318) centre (-64.3018, -10.2318) ccw
  arc A262 (-77.8018, -23.2318) -> (-77.3018, -23.7318) centre (-77.3018, -23.2318) ccw
  arc A263 (-64.3018, -23.7318) -> (-63.8018, -23.2318) centre (-64.3018, -23.2318) ccw
  line L264 (-58.2518, -9.7318) -> (-45.2518, -9.7318)
  line L265 (-58.2518, -23.7318) -> (-45.2518, -23.7318)
  line L266 (-58.7518, -10.2318) -> (-58.7518, -23.2318)
  line L267 (-44.7518, -10.2318) -> (-44.7518, -23.2318)
  arc A264 (-58.2518, -9.7318) -> (-58.7518, -10.2318) centre (-58.2518, -10.2318) ccw
  arc A265 (-44.7518, -10.2318) -> (-45.2518, -9.7318) centre (-45.2518, -10.2318) ccw
  arc A266 (-58.7518, -23.2318) -> (-58.2518, -23.7318) centre (-58.2518, -23.2318) ccw
  arc A267 (-45.2518, -23.7318) -> (-44.7518, -23.2318) centre (-45.2518, -23.2318) ccw
  line L268 (-39.2018, -9.7318) -> (-26.2018, -9.7318)
  line L269 (-39.2018, -23.7318) -> (-26.2018, -23.7318)
  line L270 (-39.7018, -10.2318) -> (-39.7018, -23.2318)
  line L271 (-25.7018, -10.2318) -> (-25.7018, -23.2318)
  arc A268 (-39.2018, -9.7318) -> (-39.7018, -10.2318) centre (-39.2018, -10.2318) ccw
  arc A269 (-25.7018, -10.2318) -> (-26.2018, -9.7318) centre (-26.2018, -10.2318) ccw
  arc A270 (-39.7018, -23.2318) -> (-39.2018, -23.7318) centre (-39.2018, -23.2318) ccw
  arc A271 (-26.2018, -23.7318) -> (-25.7018, -23.2318) centre (-26.2018, -23.2318) ccw
  line L272 (-20.1518, -9.7318) -> (-7.1518, -9.7318)
  line L273 (-20.1518, -23.7318) -> (-7.1518, -23.7318)
  line L274 (-20.6518, -10.2318) -> (-20.6518, -23.2318)
  line L275 (-6.6518, -10.2318) -> (-6.6518, -23.2318)
  arc A272 (-20.1518, -9.7318) -> (-20.6518, -10.2318) centre (-20.1518, -10.2318) ccw
  arc A273 (-6.6518, -10.2318) -> (-7.1518, -9.7318) centre (-7.1518, -10.2318) ccw
  arc A274 (-20.6518, -23.2318) -> (-20.1518, -23.7318) centre (-20.1518, -23.2318) ccw
  arc A275 (-7.1518, -23.7318) -> (-6.6518, -23.2318) centre (-7.1518, -23.2318) ccw
  line L276 (-1.1018, -9.7318) -> (11.8982, -9.7318)
  line L277 (-1.1018, -23.7318) -> (11.8982, -23.7318)
  line L278 (-1.6018, -10.2318) -> (-1.6018, -23.2318)
  line L279 (12.3982, -10.2318) -> (12.3982, -23.2318)
  arc A276 (-1.1018, -9.7318) -> (-1.6018, -10.2318) centre (-1.1018, -10.2318) ccw
  arc A277 (12.3982, -10.2318) -> (11.8982, -9.7318) centre (11.8982, -10.2318) ccw
  arc A278 (-1.6018, -23.2318) -> (-1.1018, -23.7318) centre (-1.1018, -23.2318) ccw
  arc A279 (11.8982, -23.7318) -> (12.3982, -23.2318) centre (11.8982, -23.2318) ccw
  line L280 (17.9482, -9.7318) -> (30.9482, -9.7318)
  line L281 (17.9482, -23.7318) -> (30.9482, -23.7318)
  line L282 (17.4482, -10.2318) -> (17.4482, -23.2318)
  line L283 (31.4482, -10.2318) -> (31.4482, -23.2318)
  arc A280 (17.9482, -9.7318) -> (17.4482, -10.2318) centre (17.9482, -10.2318) ccw
  arc A281 (31.4482, -10.2318) -> (30.9482, -9.7318) centre (30.9482, -10.2318) ccw
  arc A282 (17.4482, -23.2318) -> (17.9482, -23.7318) centre (17.9482, -23.2318) ccw
  arc A283 (30.9482, -23.7318) -> (31.4482, -23.2318) centre (30.9482, -23.2318) ccw
  line L284 (36.9982, -9.7318) -> (49.9982, -9.7318)
  line L285 (36.9982, -23.7318) -> (49.9982, -23.7318)
  line L286 (36.4982, -10.2318) -> (36.4982, -23.2318)
  line L287 (50.4982, -10.2318) -> (50.4982, -23.2318)
  arc A284 (36.9982, -9.7318) -> (36.4982, -10.2318) centre (36.9982, -10.2318) ccw
  arc A285 (50.4982, -10.2318) -> (49.9982, -9.7318) centre (49.9982, -10.2318) ccw
  arc A286 (36.4982, -23.2318) -> (36.9982, -23.7318) centre (36.9982, -23.2318) ccw
  arc A287 (49.9982, -23.7318) -> (50.4982, -23.2318) centre (49.9982, -23.2318) ccw
  line L288 (56.0482, -9.7318) -> (69.0482, -9.7318)
  line L289 (56.0482, -23.7318) -> (69.0482, -23.7318)
  line L290 (55.5482, -10.2318) -> (55.5482, -23.2318)
  line L291 (69.5482, -10.2318) -> (69.5482, -23.2318)
  arc A288 (56.0482, -9.7318) -> (55.5482, -10.2318) centre (56.0482, -10.2318) ccw
  arc A289 (69.5482, -10.2318) -> (69.0482, -9.7318) centre (69.0482, -10.2318) ccw
  arc A290 (55.5482, -23.2318) -> (56.0482, -23.7318) centre (56.0482, -23.2318) ccw
  arc A291 (69.0482, -23.7318) -> (69.5482, -23.2318) centre (69.0482, -23.2318) ccw
  line L292 (75.0982, -9.7318) -> (88.0982, -9.7318)
  line L293 (75.0982, -23.7318) -> (88.0982, -23.7318)
  line L294 (74.5982, -10.2318) -> (74.5982, -23.2318)
  line L295 (88.5982, -10.2318) -> (88.5982, -23.2318)
  arc A292 (75.0982, -9.7318) -> (74.5982, -10.2318) centre (75.0982, -10.2318) ccw
  arc A293 (88.5982, -10.2318) -> (88.0982, -9.7318) centre (88.0982, -10.2318) ccw
  arc A294 (74.5982, -23.2318) -> (75.0982, -23.7318) centre (75.0982, -23.2318) ccw
  arc A295 (88.0982, -23.7318) -> (88.5982, -23.2318) centre (88.0982, -23.2318) ccw
  line L296 (101.2919, -9.7318) -> (114.2919, -9.7318)
  line L297 (101.2919, -23.7318) -> (114.2919, -23.7318)
  line L298 (100.7919, -10.2318) -> (100.7919, -23.2318)
  line L299 (114.7919, -10.2318) -> (114.7919, -23.2318)
  arc A296 (101.2919, -9.7318) -> (100.7919, -10.2318) centre (101.2919, -10.2318) ccw
  arc A297 (114.7919, -10.2318) -> (114.2919, -9.7318) centre (114.2919, -10.2318) ccw
  arc A298 (100.7919, -23.2318) -> (101.2919, -23.7318) centre (101.2919, -23.2318) ccw
  arc A299 (114.2919, -23.7318) -> (114.7919, -23.2318) centre (114.2919, -23.2318) ccw
  line L300 (127.4857, -9.7318) -> (140.4857, -9.7318)
  line L301 (127.4857, -23.7318) -> (140.4857, -23.7318)
  line L302 (126.9857, -10.2318) -> (126.9857, -23.2318)
  line L303 (140.9857, -10.2318) -> (140.9857, -23.2318)
  arc A300 (127.4857, -9.7318) -> (126.9857, -10.2318) centre (127.4857, -10.2318) ccw
  arc A301 (140.9857, -10.2318) -> (140.4857, -9.7318) centre (140.4857, -10.2318) ccw
  arc A302 (126.9857, -23.2318) -> (127.4857, -23.7318) centre (127.4857, -23.2318) ccw
  arc A303 (140.4857, -23.7318) -> (140.9857, -23.2318) centre (140.4857, -23.2318) ccw
  line L304 (146.5357, -9.7318) -> (159.5357, -9.7318)
  line L305 (146.5357, -23.7318) -> (159.5357, -23.7318)
  line L306 (146.0357, -10.2318) -> (146.0357, -23.2318)
  line L307 (160.0357, -10.2318) -> (160.0357, -23.2318)
  arc A304 (146.5357, -9.7318) -> (146.0357, -10.2318) centre (146.5357, -10.2318) ccw
  arc A305 (160.0357, -10.2318) -> (159.5357, -9.7318) centre (159.5357, -10.2318) ccw
  arc A306 (146.0357, -23.2318) -> (146.5357, -23.7318) centre (146.5357, -23.2318) ccw
  arc A307 (159.5357, -23.7318) -> (160.0357, -23.2318) centre (159.5357, -23.2318) ccw
  line L308 (-136.8331, -28.7818) -> (-123.8331, -28.7818)
  line L309 (-136.8331, -42.7818) -> (-123.8331, -42.7818)
  line L310 (-137.3331, -29.2818) -> (-137.3331, -42.2818)
  line L311 (-123.3331, -29.2818) -> (-123.3331, -42.2818)
  arc A308 (-136.8331, -28.7818) -> (-137.3331, -29.2818) centre (-136.8331, -29.2818) ccw
  arc A309 (-123.3331, -29.2818) -> (-123.8331, -28.7818) centre (-123.8331, -29.2818) ccw
  arc A310 (-137.3331, -42.2818) -> (-136.8331, -42.7818) centre (-136.8331, -42.2818) ccw
  arc A311 (-123.8331, -42.7818) -> (-123.3331, -42.2818) centre (-123.8331, -42.2818) ccw
  line L312 (-113.0206, -28.7818) -> (-100.0206, -28.7818)
  line L313 (-113.0206, -42.7818) -> (-100.0206, -42.7818)
  line L314 (-113.5206, -29.2818) -> (-113.5206, -42.2818)
  line L315 (-99.5206, -29.2818) -> (-99.5206, -42.2818)
  arc A312 (-113.0206, -28.7818) -> (-113.5206, -29.2818) centre (-113.0206, -29.2818) ccw
  arc A313 (-99.5206, -29.2818) -> (-100.0206, -28.7818) centre (-100.0206, -29.2818) ccw
  arc A314 (-113.5206, -42.2818) -> (-113.0206, -42.7818) centre (-113.0206, -42.2818) ccw
  arc A315 (-100.0206, -42.7818) -> (-99.5206, -42.2818) centre (-100.0206, -42.2818) ccw
  line L316 (-89.2081, -28.7818) -> (-76.2081, -28.7818)
  line L317 (-89.2081, -42.7818) -> (-76.2081, -42.7818)
  line L318 (-89.7081, -29.2818) -> (-89.7081, -42.2818)
  line L319 (-75.7081, -29.2818) -> (-75.7081, -42.2818)
  arc A316 (-89.2081, -28.7818) -> (-89.7081, -29.2818) centre (-89.2081, -29.2818) ccw
  arc A317 (-75.7081, -29.2818) -> (-76.2081, -28.7818) centre (-76.2081, -29.2818) ccw
  arc A318 (-89.7081, -42.2818) -> (-89.2081, -42.7818) centre (-89.2081, -42.2818) ccw
  arc A319 (-76.2081, -42.7818) -> (-75.7081, -42.2818) centre (-76.2081, -42.2818) ccw
  line L320 (-17.7706, -28.7818) -> (-4.7706, -28.7818)
  line L321 (-17.7706, -42.7818) -> (-4.7706, -42.7818)
  line L322 (-18.2706, -29.2818) -> (-18.2706, -42.2818)
  line L323 (-4.2706, -29.2818) -> (-4.2706, -42.2818)
  arc A320 (-17.7706, -28.7818) -> (-18.2706, -29.2818) centre (-17.7706, -29.2818) ccw
  arc A321 (-4.2706, -29.2818) -> (-4.7706, -28.7818) centre (-4.7706, -29.2818) ccw
  arc A322 (-18.2706, -42.2818) -> (-17.7706, -42.7818) centre (-17.7706, -42.2818) ccw
  arc A323 (-4.7706, -42.7818) -> (-4.2706, -42.2818) centre (-4.7706, -42.2818) ccw
  line L324 (-64.2706, -29.7818) -> (-58.2706, -29.7818)
  line L325 (-64.2706, -44.7818) -> (-58.2706, -44.7818)
  line L326 (-64.7706, -30.2818) -> (-64.7706, -44.2818)
  line L327 (-57.7706, -30.2818) -> (-57.7706, -44.2818)
  arc A324 (-64.2706, -29.7818) -> (-64.7706, -30.2818) centre (-64.2706, -30.2818) ccw
  arc A325 (-57.7706, -30.2818) -> (-58.2706, -29.7818) centre (-58.2706, -30.2818) ccw
  arc A326 (-64.7706, -44.2818) -> (-64.2706, -44.7818) centre (-64.2706, -44.2818) ccw
  arc A327 (-58.2706, -44.7818) -> (-57.7706, -44.2818) centre (-58.2706, -44.2818) ccw
  line L328 (35.7294, -29.7818) -> (41.7294, -29.7818)
  line L329 (35.7294, -44.7818) -> (41.7294, -44.7818)
  line L330 (35.2294, -30.2818) -> (35.2294, -44.2818)
  line L331 (42.2294, -30.2818) -> (42.2294, -44.2818)
  arc A328 (35.7294, -29.7818) -> (35.2294, -30.2818) centre (35.7294, -30.2818) ccw
  arc A329 (42.2294, -30.2818) -> (41.7294, -29.7818) centre (41.7294, -30.2818) ccw
  arc A330 (35.2294, -44.2818) -> (35.7294, -44.7818) centre (35.7294, -44.2818) ccw
  arc A331 (41.7294, -44.7818) -> (42.2294, -44.2818) centre (41.7294, -44.2818) ccw
  line L332 (51.2857, -28.7818) -> (64.2857, -28.7818)
  line L333 (51.2857, -42.7818) -> (64.2857, -42.7818)
  line L334 (50.7857, -29.2818) -> (50.7857, -42.2818)
  line L335 (64.7857, -29.2818) -> (64.7857, -42.2818)
  arc A332 (51.2857, -28.7818) -> (50.7857, -29.2818) centre (51.2857, -29.2818) ccw
  arc A333 (64.7857, -29.2818) -> (64.2857, -28.7818) centre (64.2857, -29.2818) ccw
  arc A334 (50.7857, -42.2818) -> (51.2857, -42.7818) centre (51.2857, -42.2818) ccw
  arc A335 (64.2857, -42.7818) -> (64.7857, -42.2818) centre (64.2857, -42.2818) ccw
  line L336 (70.3357, -28.7818) -> (83.3357, -28.7818)
  line L337 (70.3357, -42.7818) -> (83.3357, -42.7818)
  line L338 (69.8357, -29.2818) -> (69.8357, -42.2818)
  line L339 (83.8357, -29.2818) -> (83.8357, -42.2818)
  arc A336 (70.3357, -28.7818) -> (69.8357, -29.2818) centre (70.3357, -29.2818) ccw
  arc A337 (83.8357, -29.2818) -> (83.3357, -28.7818) centre (83.3357, -29.2818) ccw
  arc A338 (69.8357, -42.2818) -> (70.3357, -42.7818) centre (70.3357, -42.2818) ccw
  arc A339 (83.3357, -42.7818) -> (83.8357, -42.2818) centre (83.3357, -42.2818) ccw
  line L340 (89.3857, -28.7818) -> (102.3857, -28.7818)
  line L341 (89.3857, -42.7818) -> (102.3857, -42.7818)
  line L342 (88.8857, -29.2818) -> (88.8857, -42.2818)
  line L343 (102.8857, -29.2818) -> (102.8857, -42.2818)
  arc A340 (89.3857, -28.7818) -> (88.8857, -29.2818) centre (89.3857, -29.2818) ccw
  arc A341 (102.8857, -29.2818) -> (102.3857, -28.7818) centre (102.3857, -29.2818) ccw
  arc A342 (88.8857, -42.2818) -> (89.3857, -42.7818) centre (89.3857, -42.2818) ccw
  arc A343 (102.3857, -42.7818) -> (102.8857, -42.2818) centre (102.3857, -42.2818) ccw
  line L344 (108.4357, -28.7818) -> (121.4357, -28.7818)
  line L345 (108.4357, -42.7818) -> (121.4357, -42.7818)
  line L346 (107.9357, -29.2818) -> (107.9357, -42.2818)
  line L347 (121.9357, -29.2818) -> (121.9357, -42.2818)
  arc A344 (108.4357, -28.7818) -> (107.9357, -29.2818) centre (108.4357, -29.2818) ccw
  arc A345 (121.9357, -29.2818) -> (121.4357, -28.7818) centre (121.4357, -29.2818) ccw
  arc A346 (107.9357, -42.2818) -> (108.4357, -42.7818) centre (108.4357, -42.2818) ccw
  arc A347 (121.4357, -42.7818) -> (121.9357, -42.2818) centre (121.4357, -42.2818) ccw
  line L348 (127.4857, -28.7818) -> (140.4857, -28.7818)
  line L349 (127.4857, -42.7818) -> (140.4857, -42.7818)
  line L350 (126.9857, -29.2818) -> (126.9857, -42.2818)
  line L351 (140.9857, -29.2818) -> (140.9857, -42.2818)
  arc A348 (127.4857, -28.7818) -> (126.9857, -29.2818) centre (127.4857, -29.2818) ccw
  arc A349 (140.9857, -29.2818) -> (140.4857, -28.7818) centre (140.4857, -29.2818) ccw
  arc A350 (126.9857, -42.2818) -> (127.4857, -42.7818) centre (127.4857, -42.2818) ccw
  arc A351 (140.4857, -42.7818) -> (140.9857, -42.2818) centre (140.4857, -42.2818) ccw
  line L352 (146.5357, -28.7818) -> (159.5357, -28.7818)
  line L353 (146.5357, -42.7818) -> (159.5357, -42.7818)
  line L354 (146.0357, -29.2818) -> (146.0357, -42.2818)
  line L355 (160.0357, -29.2818) -> (160.0357, -42.2818)
  arc A352 (146.5357, -28.7818) -> (146.0357, -29.2818) centre (146.5357, -29.2818) ccw
  arc A353 (160.0357, -29.2818) -> (159.5357, -28.7818) centre (159.5357, -29.2818) ccw
  arc A354 (146.0357, -42.2818) -> (146.5357, -42.7818) centre (146.5357, -42.2818) ccw
  arc A355 (159.5357, -42.7818) -> (160.0357, -42.2818) centre (159.5357, -42.2818) ccw
  line L356 (-153.6501, 86.0492) -> (212.5639, 86.0492)
  line L357 (212.5639, 86.0492) -> (212.5639, -64.1628)
  line L358 (212.5639, -64.1628) -> (-153.6501, -64.1628)